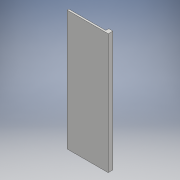
# Autodesk Inventor part: base
Saved by Autodesk Inventor 2018.2 (Build 222227000, 227)
## iProperties
Created: 2018-01-31
Part Number: base
Material: Generic
Document SubType Name: Modeling
Designer: wharr
Density: 1 g/cm^3
Appearance: Default
Author: wharr
Autodesk Inventor part; units mm, degrees
ref_plane "YZ Plane" through (0, 0, 0) normal (1, 0, 0) x (0, 1, 0)
ref_plane "XZ Plane" through (0, 0, 0) normal (0, 1, 0) x (-1, 0, 0)
ref_plane "XY Plane" through (0, 0, 0) normal (0, 0, 1) x (1, 0, 0)
sketch "Sketch1" plane through (0, 0, 0) normal (0, 1, 0) x (-1, 0, 0)
  line L0 (-35, 102.5) -> (35, 102.5)
  line L1 (35, 102.5) -> (35, -102.5)
  line L2 (35, -102.5) -> (-35, -102.5)
  line L3 (-35, -102.5) -> (-35, 102.5)
  line L4 (-35, 102.5) -> (35, -102.5) construction
  line L5 (35, 102.5) -> (-35, -102.5) construction
  point P0 (0, 0)
  dimension "d0" = 205
  dimension "d1" = 70
  constraints: 12 end point, 2 midpoint, 2 parallel, 1 horizontal, 1 perpendicular
  measures "d0" distance of L0.end L1.end
  measures "d1" distance of L1.end L2.end
extrude "Extrusion1" add sketch "Sketch1" along normal blind 3
sketch "Sketch2" plane through (0, 3, 0) normal (0, 1, 0) x (1, 0, 0)
  line L0 (-35, -102.5) -> (35, -102.5) projected
  line L1 (35, 102.5) -> (-35, 102.5) projected
  line L2 (35, -102.5) -> (28, -102.5)
  line L3 (28, -102.5) -> (28, 102.5)
  line L4 (28, 102.5) -> (35, 102.5)
  line L5 (35, 102.5) -> (35, -102.5)
  line L6 (30, 100.5) -> (30, -100.5)
  line L7 (30, -100.5) -> (33, -100.5)
  line L8 (33, -100.5) -> (33, 100.5)
  line L9 (33, 100.5) -> (30, 100.5)
  point P0 (0, 0)
  dimension "d4" = 7
  dimension "d5" = 2
  constraints: 16 end point, 4 parallel, 2 perpendicular, 1 horizontal, 1 point on line, 3 other
  measures "d4" distance between parallel lines of L5 L3
  measures "d5" distance between parallel lines of L3 L6
extrude "Extrusion2" add sketch "Sketch2" along normal blind 5
body "Solid1"
